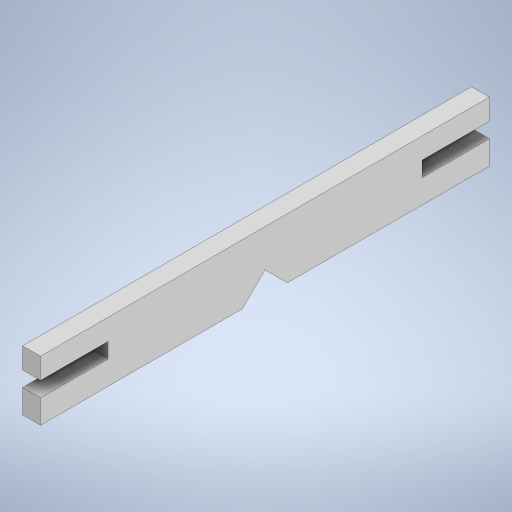
# Autodesk Inventor part: insert spacer - v1
Saved by Autodesk Inventor 2023 (Build 270158000, 158)
## iProperties
Created: 2022-07-08
Part Number: insert spacer - v1
Material: Generic
Document SubType Name: Modeling
Designer: Caleb
Density: 1 g/cm^3
Appearance: Default
Author: Caleb
Autodesk Inventor part; units mm, degrees
ref_plane "YZ Plane" through (0, 0, 0) normal (1, 0, 0) x (0, 1, 0)
ref_plane "XZ Plane" through (0, 0, 0) normal (0, 1, 0) x (-1, 0, 0)
ref_plane "XY Plane" through (0, 0, 0) normal (0, 0, 1) x (1, 0, 0)
sketch "Sketch1" plane through (0, 0, 0) normal (1, 0, 0) x (0, 1, 0)
  line L0 (-1, -7.5) -> (1, -7.5)
  line L1 (1, -7.5) -> (1, 7.5)
  line L2 (1, 7.5) -> (-1, 7.5)
  line L3 (-1, 7.5) -> (-1, -7.5)
  line L4 (-1, -7.5) -> (1, 7.5) construction
  line L5 (1, -7.5) -> (-1, 7.5) construction
  point P0 (0, 0)
  dimension "d0" = 2
  dimension "d1" = 15
  constraints: 12 end point, 2 midpoint, 2 parallel, 1 horizontal, 1 perpendicular
  measures "d0" distance of L1.end L2.end
  measures "d1" distance of L0.end L1.end
extrude "Extrusion1" add sketch "Sketch1" along normal blind 0.6
sketch "Sketch2" plane through (0.6, 0, 0) normal (1, 0, 0) x (0, 0, -1)
  line L0 (-7.5, 1) -> (-7.5, -1) projected
  line L1 (-7.5, 0.3) -> (-5.25, 0.3)
  line L2 (-5.25, 0.3) -> (-5.25, -0.2)
  line L3 (-5.25, -0.2) -> (-7.5, -0.2)
  line L4 (-7.5, -0.2) -> (-7.5, 0.3)
  line L5 (0, 1.1867) -> (0, -1.275)
  line L6 (7.5, 1) -> (7.5, -1)
  line L7 (7.5, 0.3) -> (5.25, 0.3)
  line L8 (5.25, 0.3) -> (5.25, -0.2)
  line L9 (5.25, -0.2) -> (7.5, -0.2)
  line L10 (7.5, -0.2) -> (7.5, 0.3)
  line L11 (7.5, 1) -> (-7.5, 1) projected
  point P0 (0, 0)
  dimension "d4" = 0.5
  dimension "d9" = 0.7
  dimension "d15" = 10.5
  constraints: 20 end point, 6 symmetric about line, 2 parallel, 2 point on line, 1 horizontal, 1 perpendicular, 1 vertical
  measures "d4" distance of L1.end L2.end
  measures "d9" distance between parallel lines of L11 L1
  measures "d15" distance between parallel lines of L8 L2
extrude "Extrusion2" cut sketch "Sketch2" against normal blind 0.6
sketch "Sketch3" plane through (0.6, 0, 0) normal (1, 0, 0) x (0, 0, -1)
  line L0 (-7.5, -1) -> (7.5, -1) projected
  line L1 (-0.75, -1) -> (0, -0.25)
  line L2 (0, -0.25) -> (0.75, -1)
  point P0 (0, 0)
  dimension "d10" = 45
  dimension "d11" = 45
  dimension "d12" = 1.5
  constraints: 4 end point, 2 point on line, 1 vertical alignment
  measures "d10" angle of L0 L1
  measures "d11" angle of L0 L2
  measures "d12" distance of L1.start L2.end
extrude "Extrusion3" cut sketch "Sketch3" against normal blind 0.6
equation "\"d11\" = d10"
body "Solid1"
